Autodesk Inventor part; units mm, degrees
(part 3 of 3)
  line L1891 (2.3516, 3.9753) -> (2.3994, 4.0491)
  line L1892 (2.3994, 4.0491) -> (2.4275, 4.0862)
  line L1893 (2.4275, 4.0862) -> (2.4785, 4.1429)
  line L1894 (2.4785, 4.1429) -> (2.5137, 4.1777)
  line L1895 (2.5137, 4.1777) -> (2.5571, 4.2171)
  line L1896 (2.5571, 4.2171) -> (2.609, 4.2604)
  line L1897 (2.609, 4.2604) -> (2.6681, 4.3057)
  line L1898 (2.6681, 4.3057) -> (2.7371, 4.3541)
  line L1899 (2.7371, 4.3541) -> (2.8135, 4.403)
  line L1900 (2.8135, 4.403) -> (2.9006, 4.4538)
  line L1901 (2.9006, 4.4538) -> (2.9964, 4.5044)
  line L1902 (2.9964, 4.5044) -> (3.0907, 4.5494)
  arc A39 (3.3717, 4.3453) -> (3.0907, 4.5494) centre (0, 0) ccw
  line L1903 (3.3717, 4.3453) -> (3.358, 4.2416)
  line L1904 (3.358, 4.2416) -> (3.3395, 4.1349)
  line L1905 (3.3395, 4.1349) -> (3.3181, 4.0364)
  line L1906 (3.3181, 4.0364) -> (3.2952, 3.9486)
  line L1907 (3.2952, 3.9486) -> (3.2704, 3.868)
  line L1908 (3.2704, 3.868) -> (3.2457, 3.7978)
  line L1909 (3.2457, 3.7978) -> (3.2205, 3.7351)
  line L1910 (3.2205, 3.7351) -> (3.1965, 3.6817)
  line L1911 (3.1965, 3.6817) -> (3.1743, 3.6374)
  line L1912 (3.1743, 3.6374) -> (3.1361, 3.5714)
  line L1913 (3.1361, 3.5714) -> (3.1095, 3.5332)
  line L1914 (3.1095, 3.5332) -> (3.0541, 3.465)
  line L1915 (3.0541, 3.465) -> (3.0213, 3.4148)
  line L1916 (3.0213, 3.4148) -> (3.0084, 3.391)
  line L1917 (3.0084, 3.391) -> (2.9979, 3.3682)
  line L1918 (2.9979, 3.3682) -> (2.9895, 3.3465)
  line L1919 (2.9895, 3.3465) -> (2.9834, 3.326)
  line L1920 (2.9834, 3.326) -> (2.9794, 3.3067)
  line L1921 (2.9794, 3.3067) -> (2.9775, 3.2887)
  line L1922 (2.9775, 3.2887) -> (2.9777, 3.2722)
  line L1923 (2.9777, 3.2722) -> (2.9798, 3.2571)
  line L1924 (2.9798, 3.2571) -> (2.9838, 3.2436)
  line L1925 (2.9838, 3.2436) -> (2.9896, 3.2317)
  line L1926 (2.9896, 3.2317) -> (3.0017, 3.2171)
  line L1927 (3.0017, 3.2171) -> (3.1113, 3.1113)
  line L1928 (3.1113, 3.1113) -> (3.2171, 3.0017)
  line L1929 (3.2171, 3.0017) -> (3.2317, 2.9896)
  line L1930 (3.2317, 2.9896) -> (3.2436, 2.9838)
  line L1931 (3.2436, 2.9838) -> (3.2571, 2.9798)
  line L1932 (3.2571, 2.9798) -> (3.2722, 2.9777)
  line L1933 (3.2722, 2.9777) -> (3.2887, 2.9775)
  line L1934 (3.2887, 2.9775) -> (3.3067, 2.9794)
  line L1935 (3.3067, 2.9794) -> (3.326, 2.9834)
  line L1936 (3.326, 2.9834) -> (3.3465, 2.9895)
  line L1937 (3.3465, 2.9895) -> (3.3682, 2.9979)
  line L1938 (3.3682, 2.9979) -> (3.391, 3.0084)
  line L1939 (3.391, 3.0084) -> (3.4148, 3.0213)
  line L1940 (3.4148, 3.0213) -> (3.465, 3.0541)
  line L1941 (3.465, 3.0541) -> (3.5332, 3.1095)
  line L1942 (3.5332, 3.1095) -> (3.5714, 3.1361)
  line L1943 (3.5714, 3.1361) -> (3.6374, 3.1743)
  line L1944 (3.6374, 3.1743) -> (3.6817, 3.1965)
  line L1945 (3.6817, 3.1965) -> (3.7351, 3.2205)
  line L1946 (3.7351, 3.2205) -> (3.7978, 3.2457)
  line L1947 (3.7978, 3.2457) -> (3.868, 3.2704)
  line L1948 (3.868, 3.2704) -> (3.9486, 3.2952)
  line L1949 (3.9486, 3.2952) -> (4.0364, 3.3181)
  line L1950 (4.0364, 3.3181) -> (4.1349, 3.3395)
  line L1951 (4.1349, 3.3395) -> (4.2416, 3.358)
  line L1952 (4.2416, 3.358) -> (4.3453, 3.3717)
  arc A40 (4.5494, 3.0907) -> (4.3453, 3.3717) centre (0, 0) ccw
  line L1953 (4.5494, 3.0907) -> (4.5044, 2.9964)
  line L1954 (4.5044, 2.9964) -> (4.4538, 2.9006)
  line L1955 (4.4538, 2.9006) -> (4.403, 2.8135)
  line L1956 (4.403, 2.8135) -> (4.3541, 2.7371)
  line L1957 (4.3541, 2.7371) -> (4.3057, 2.6681)
  line L1958 (4.3057, 2.6681) -> (4.2604, 2.609)
  line L1959 (4.2604, 2.609) -> (4.2171, 2.5571)
  line L1960 (4.2171, 2.5571) -> (4.1777, 2.5137)
  line L1961 (4.1777, 2.5137) -> (4.1429, 2.4785)
  line L1962 (4.1429, 2.4785) -> (4.0862, 2.4275)
  line L1963 (4.0862, 2.4275) -> (4.0491, 2.3994)
  line L1964 (4.0491, 2.3994) -> (3.9753, 2.3516)
  line L1965 (3.9753, 2.3516) -> (3.9286, 2.314)
  line L1966 (3.9286, 2.314) -> (3.9091, 2.2954)
  line L1967 (3.9091, 2.2954) -> (3.892, 2.277)
  line L1968 (3.892, 2.277) -> (3.8773, 2.2589)
  line L1969 (3.8773, 2.2589) -> (3.8652, 2.2413)
  line L1970 (3.8652, 2.2413) -> (3.8554, 2.2242)
  line L1971 (3.8554, 2.2242) -> (3.8481, 2.2077)
  line L1972 (3.8481, 2.2077) -> (3.8431, 2.1919)
  line L1973 (3.8431, 2.1919) -> (3.8404, 2.1769)
  line L1974 (3.8404, 2.1769) -> (3.8401, 2.1628)
  line L1975 (3.8401, 2.1628) -> (3.842, 2.1497)
  line L1976 (3.842, 2.1497) -> (3.8489, 2.1321)
  line L1977 (3.8489, 2.1321) -> (3.9204, 1.9976)
  line L1978 (3.9204, 1.9976) -> (3.9872, 1.8607)
  line L1979 (3.9872, 1.8607) -> (3.9974, 1.8447)
  line L1980 (3.9974, 1.8447) -> (4.0069, 1.8354)
  line L1981 (4.0069, 1.8354) -> (4.0185, 1.8274)
  line L1982 (4.0185, 1.8274) -> (4.0322, 1.8208)
  line L1983 (4.0322, 1.8208) -> (4.0479, 1.8155)
  line L1984 (4.0479, 1.8155) -> (4.0655, 1.8118)
  line L1985 (4.0655, 1.8118) -> (4.0851, 1.8096)
  line L1986 (4.0851, 1.8096) -> (4.1065, 1.8091)
  line L1987 (4.1065, 1.8091) -> (4.1297, 1.8103)
  line L1988 (4.1297, 1.8103) -> (4.1547, 1.8133)
  line L1989 (4.1547, 1.8133) -> (4.1813, 1.8182)
  line L1990 (4.1813, 1.8182) -> (4.2391, 1.8339)
  line L1991 (4.2391, 1.8339) -> (4.3212, 1.8655)
  line L1992 (4.3212, 1.8655) -> (4.3657, 1.879)
  line L1993 (4.3657, 1.879) -> (4.4403, 1.8949)
  line L1994 (4.4403, 1.8949) -> (4.4892, 1.9023)
  line L1995 (4.4892, 1.9023) -> (4.5475, 1.9087)
  line L1996 (4.5475, 1.9087) -> (4.6149, 1.9132)
  line L1997 (4.6149, 1.9132) -> (4.6893, 1.9151)
  line L1998 (4.6893, 1.9151) -> (4.7736, 1.9137)
  line L1999 (4.7736, 1.9137) -> (4.8642, 1.9084)
  line L2000 (4.8642, 1.9084) -> (4.9645, 1.8983)
  line L2001 (4.9645, 1.8983) -> (5.0717, 1.8829)
  line L2002 (5.0717, 1.8829) -> (5.1745, 1.8639)
  arc A41 (5.2818, 1.5336) -> (5.1745, 1.8639) centre (0, 0) ccw
  line L2003 (5.2818, 1.5336) -> (5.2098, 1.4578)
  line L2004 (5.1322, 1.3823) -> (5.0569, 1.3152)
  line L2005 (-1.4578, 5.2098) -> (-1.3823, 5.1322)
  point P0 (1.118, 1)
  point P1 (-1.118, 1)
  point P2 (5.2818, 1.5336)
  point P3 (5.1745, 1.8639)
  point P4 (4.5494, 3.0907)
  point P5 (4.3453, 3.3717)
  point P6 (3.3717, 4.3453)
  point P7 (3.0907, 4.5494)
  point P8 (1.8639, 5.1745)
  point P9 (1.5336, 5.2818)
  point P10 (0.1736, 5.4973)
  point P11 (-0.1736, 5.4973)
  point P12 (-1.5336, 5.2818)
  point P13 (-1.8639, 5.1745)
  point P14 (-3.0907, 4.5494)
  point P15 (-3.3717, 4.3453)
  point P16 (-4.3453, 3.3717)
  point P17 (-4.5494, 3.0907)
  point P18 (-5.1745, 1.8639)
  point P19 (-5.2818, 1.5336)
  point P20 (-5.4973, 0.1736)
  point P21 (-5.4973, -0.1736)
  point P22 (-5.2818, -1.5336)
  point P23 (-5.1745, -1.8639)
  point P24 (-4.5494, -3.0907)
  point P25 (-4.3453, -3.3717)
  point P26 (-3.3717, -4.3453)
  point P27 (-3.0907, -4.5494)
  point P28 (-1.8639, -5.1745)
  point P29 (-1.5336, -5.2818)
  point P30 (-0.1736, -5.4973)
  point P31 (0.1736, -5.4973)
  point P32 (1.5336, -5.2818)
  point P33 (1.8639, -5.1745)
  point P34 (3.0907, -4.5494)
  point P35 (3.3717, -4.3453)
  point P36 (4.3453, -3.3717)
  point P37 (4.5494, -3.0907)
  point P38 (5.1745, -1.8639)
  point P39 (5.2818, -1.5336)
  point P40 (5.4973, -0.1736)
  point P41 (5.4973, 0.1736)
  constraints: 4012 end point, 84 point on circle, 42 centre point
extrude "Extrusion1" add sketch "Sketch2" against normal blind 3
sketch "Sketch3" plane through (0, 0, -3) normal (0, 0, -1) x (-1, 0, 0)
  circle A0 centre (0, 0) radius 1.55
  line L0 (1.118, 1) -> (-1.118, 1)
  line L1 (0, 1) -> (0, 1.05)
  line L2 (0, 1.05) -> (-1.1402, 1.05)
  line L3 (0, 1.05) -> (1.1402, 1.05)
  dimension "d2" = 3.1
  dimension "d4" = 0.05
  constraints: 6 end point, 2 point on circle, 1 centre point, 1 coincident, 1 midpoint, 1 perpendicular, 1 point on line, 1 vertical
  measures "d2" diameter of A0
  measures "d4" distance of L1.start L1.end
extrude "Extrusion2" cut sketch "Sketch3" against normal blind 10 contours A0 L2 L3 picked at (-0.008, -0.6757)
body "Solid1"
